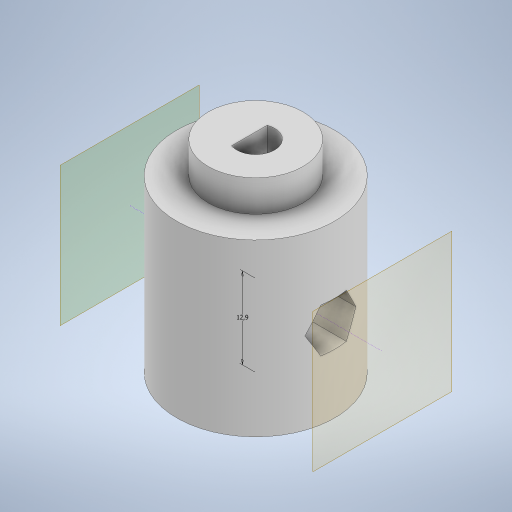
# Autodesk Inventor part: StuurPotentiometerConnector3.0
Saved by Autodesk Inventor 2024 (Build 280153000, 153)
## iProperties
Created: 2023-11-20
Part Number: StuurPotentiometerConnector3.0
Material: Generic
Document SubType Name: Modeling
Designer: Nikita
Density: 1 g/cm^3
Appearance: Default
Author: Nikita
Autodesk Inventor part; units mm, degrees
ref_plane "YZ Plane" through (0, 0, 0) normal (1, 0, 0) x (0, 1, 0)
ref_plane "XZ Plane" through (0, 0, 0) normal (0, 1, 0) x (-1, 0, 0)
ref_plane "XY Plane" through (0, 0, 0) normal (0, 0, 1) x (1, 0, 0)
sketch "Sketch1" plane through (0, 0, 0) normal (0, 1, 0) x (-1, 0, 0)
  circle A0 centre (0, 0) radius 12.5
  dimension "d0" = 25
  constraints: 1 centre point, 1 coincident
  measures "d0" diameter of A0
extrude "Extrusion1" add sketch "Sketch1" along normal blind 27
sketch "Sketch2" plane through (0, 27, 0) normal (0, 1, 0) x (1, 0, 0)
  circle A0 centre (0, 0) radius 7.5
  arc A1 (-1, -2.8284) -> (-1, 2.8284) centre (0, 0) ccw
  line L0 (3, 0) -> (-1, 0) construction
  line L1 (-1, 0) -> (-1, 2.8284) construction
  line L2 (-1, 2.8284) -> (-1, -2.8284)
  dimension "d4" = 15
  dimension "d5" = 6
  dimension "d6" = 4
  constraints: 6 end point, 3 point on circle, 2 centre point, 2 coincident, 1 horizontal, 1 perpendicular, 1 vertical
  measures "d4" diameter of A0
  measures "d5" diameter of A1
  measures "d6" distance of L0.start L0.end
extrude "Extrusion2" add sketch "Sketch2" along normal blind 5
sketch "Sketch3" plane through (0, 0, 0) normal (0, -1, 0) x (1, 0, 0)
  circle A0 centre (0, 0) radius 5.25
  dimension "d9" = 10.5
  constraints: 1 centre point, 1 coincident
  measures "d9" diameter of A0
extrude "Extrusion3" cut sketch "Sketch3" against normal blind 25
sketch "Sketch6" plane through (0, 0, 0) normal (0, 0, 1) x (1, 0, 0)
  line L0 (0, 12.9265) -> (-19.9756, 12.9265) construction
  line L1 (0, 12.9265) -> (20.0738, 12.9265) construction
  line L2 (0, 0) -> (0, 12.9) construction
  dimension "d19" = 12.9
  constraints: 6 end point, 2 horizontal, 1 vertical
  measures "d19" distance of L2.start L2.end
ref_plane "Work Plane1" through (-19.9756, 12.9265, 0) normal (-1, 0, 0) x (0, -1, 0)
sketch "Sketch7" plane through (-19.9756, 12.9265, 0) normal (-1, 0, 0) x (0, -1, 0)
  circle A0 centre (0, 0) radius 4
  point P0 (12.9265, 0)
  dimension "d16" = 8
  constraints: 1 centre point
  measures "d16" diameter of A0
extrude "Extrusion5" cut sketch "Sketch7" against normal blind 10
ref_plane "Work Plane2" through (20.0738, 12.9265, 0) normal (1, 0, 0) x (0, 1, 0)
sketch "Sketch8" plane through (20.0738, 12.9265, 0) normal (1, 0, 0) x (0, 1, 0)
  line L0 (-3.5, -2.0207) -> (-3.5, 2.0207)
  line L1 (-3.5, 2.0207) -> (0, 4.0415)
  line L2 (0, 4.0415) -> (3.5, 2.0207)
  line L3 (3.5, 2.0207) -> (3.5, -2.0207)
  line L4 (3.5, -2.0207) -> (0, -4.0415)
  line L5 (0, -4.0415) -> (-3.5, -2.0207)
  point P0 (-12.9265, 0)
  point P1 (0, 0)
  constraints: 12 end point, 1 vertical, 13 other
extrude "Extrusion6" cut sketch "Sketch8" against normal blind 17.9375
sketch "Sketch9" plane through (-19.9756, 12.9265, 0) normal (-1, 0, 0) x (0, -1, 0)
  circle A0 centre (0, 0) radius 2.25
  point P0 (12.9265, 0)
  dimension "d22" = 4.5
  constraints: 1 centre point
  measures "d22" diameter of A0
extrude "Extrusion7" cut sketch "Sketch9" against normal blind 17.9375
body "Solid1"
